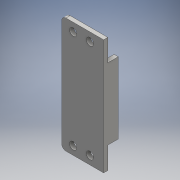
# Autodesk Inventor part: SwitchMountTop
Saved by Autodesk Inventor 2016 (Build 200138000, 138)
## iProperties
Created: 2026-04-05
Part Number: SwitchMountTop
Material: Generic
Document SubType Name: Modeling
Designer: Steve
Density: 1 g/cm^3
Appearance: Default
Author: Steve
Autodesk Inventor part; units mm, degrees
ref_plane "YZ Plane" through (0, 0, 0) normal (1, 0, 0) x (0, 1, 0)
ref_plane "XZ Plane" through (0, 0, 0) normal (0, 1, 0) x (-1, 0, 0)
ref_plane "XY Plane" through (0, 0, 0) normal (0, 0, 1) x (1, 0, 0)
sketch "Sketch1" plane through (0, 0, 0) normal (0, 1, 0) x (-1, 0, 0)
  line L0 (10.352, 30.898) -> (-9.648, 30.898)
  line L1 (-9.648, 30.898) -> (-9.648, -24.102)
  line L2 (-9.648, -24.102) -> (10.352, -24.102)
  line L3 (10.352, -24.102) -> (10.352, 30.898)
  circle A0 centre (4.852, 26.898) radius 1.75
  circle A1 centre (-3.148, 26.898) radius 1.75
  circle A2 centre (4.852, -20.102) radius 1.75
  circle A3 centre (-3.148, -20.102) radius 1.75
  point P0 (0, 0)
  dimension "d0" = 55
  dimension "d1" = 20
  dimension "d2" = 3.5
  dimension "d3" = 3.5
  dimension "d4" = 3.5
  dimension "d5" = 3.5
  dimension "d6" = 4
  dimension "d7" = 4
  dimension "d8" = 4
  dimension "d9" = 4
  dimension "d10" = 5.5
  dimension "d11" = 8
  dimension "d12" = 5.5
  dimension "d13" = 8
  constraints: 8 end point, 4 centre point, 2 parallel, 1 horizontal, 1 perpendicular
  measures "d0" distance of L2.end L0.start
  measures "d1" distance of L1.end L2.end
  measures "d2" diameter of A0
  measures "d3" diameter of A1
  measures "d4" diameter of A2
  measures "d5" diameter of A3
  measures "d6" distance from line of L0 A0.centre
  measures "d7" distance from line of L0 A1.centre
  measures "d8" distance from line of L2 A3.centre
  measures "d9" distance from line of L2 A2.centre
  measures "d10" distance from line of L3 A2.centre
  measures "d11" distance of A3.centre A2.centre
  measures "d12" distance from line of L3 A0.centre
  measures "d13" distance of A1.centre A0.centre
extrude "Extrusion1" add sketch "Sketch1" along normal blind 2
sketch "Sketch2" plane through (0, 2, 0) normal (0, 1, 0) x (1, 0, 0)
  line L0 (9.648, -30.898) -> (9.648, 24.102) projected
  line L1 (9.648, -20.398) -> (7.648, -20.398)
  line L2 (7.648, -20.398) -> (7.648, 13.602)
  line L3 (7.648, 13.602) -> (9.648, 13.602)
  line L4 (9.648, 13.602) -> (9.648, -20.398)
  line L5 (-10.352, -30.898) -> (9.648, -30.898) projected
  line L6 (9.648, 24.102) -> (-10.352, 24.102) projected
  point P0 (0, 0)
  dimension "d16" = 2
  dimension "d17" = 34
  dimension "d18" = 10.5
  dimension "d19" = 10.5
  constraints: 8 end point, 2 parallel, 1 horizontal, 1 perpendicular, 1 point on line
  measures "d16" distance of L2.end L3.end
  measures "d17" distance of L1.end L2.end
  measures "d18" distance between parallel lines of L5 L1
  measures "d19" distance between parallel lines of L6 L3
extrude "Extrusion2" add sketch "Sketch2" along normal blind 5
fillet "Fillet1" radius 2 2 edges at (-10.352, 1, 30.898) (-10.352, 1, -24.102)
body "Solid1"
